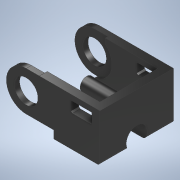
# Autodesk Inventor part: X-linear bearing shroud left half
Saved by Autodesk Inventor 2020.4 (Build 244396000, 396)
## iProperties
Created: 2021-02-25
Part Number: X-linear bearing shroud left half
Material: ABS Plastic
Document SubType Name: Modeling
Designer: AOB
Surface Area: 41.2852 cm^2
Density: 1.06 g/cm^3
Appearance: Glossy - Black
Mass: 4.81018 g
Volume: 4.53791 cm^3
Author: AOB
Autodesk Inventor part; units mm, degrees
ref_plane "YZ Plane" through (0, 0, 0) normal (1, 0, 0) x (0, 1, 0)
ref_plane "XZ Plane" through (0, 0, 0) normal (0, 1, 0) x (-1, 0, 0)
sketch "Sketch1" plane through (0, 0, 0) normal (0, 0, 1) x (1, 0, 0)
  line L0 (5.0224, 7.5) -> (28, 7.5)
  line L1 (5.0224, 7.5) -> (5.7962, 7.5)
  arc A0 (0, 7.5) -> (-0.0125, -7.5) centre (0, 0) ccw
  line L2 (5.0224, 7.5) -> (0, 7.5)
  line L3 (23.4991, -10.4606) -> (10.5, -10.4606)
  line L4 (10.5, -10.4606) -> (10.5, -7.5)
  line L5 (17.5, 1.4713) -> (24.5, 1.4713)
  line L6 (25, 1.9713) -> (25, 5.5001)
  line L7 (28, 7.5001) -> (28, -9.4606)
  line L8 (27, -10.4606) -> (23.4991, -10.4606)
  arc A1 (27, -10.4606) -> (28, -9.4606) centre (27, -9.4606) ccw
  line L9 (24.5, 1.4713) -> (25, 1.9713)
  line L10 (17.5, 1.4713) -> (17, 1.9713)
  line L11 (10.5, -7.5) -> (-0.0125, -7.5)
  line L12 (25, 5.5001) -> (17, 5.5001)
  line L13 (17, 7.5001) -> (17, 7.5)
  line L14 (17, 5.5001) -> (17, 1.9713)
  point P0 (25, 1.4713)
  point P1 (17, 1.4713)
  dimension "d58" = 1
  dimension "d70" = 28
  dimension "d71" = 17.5
  constraints: 30 end point, 6 perpendicular, 6 point on line, 4 horizontal, 4 point on circle, 3 tangent, 2 centre point, 1 coincident, 1 vertical
  measures "d58" radius of A1
  measures "d70" distance from line of L7 point (0, 0)
  measures "d71" distance between parallel lines of L7 L4
extrude "Extrusion1" add sketch "Sketch1" along normal blind 3
sketch "Sketch3" plane through (0, 0, 0) normal (0, 0, -1) x (-1, 0, 0)
  line L0 (-10.5, -10.4606) -> (-27, -10.4606)
  line L1 (-10.5, -7.5) -> (-10.5, -10.4606)
  arc A0 (-28, -9.4606) -> (-27, -10.4606) centre (-27, -9.4606) ccw
  line L2 (-28, -9.4606) -> (-28, 7.5)
  line L3 (-25, 5.5001) -> (-25, 1.9713)
  line L4 (-28, 7.5) -> (-25, 7.5)
  line L5 (-25, 5.5001) -> (-25, 7.5)
  line L6 (-25, 1.9713) -> (-24.5, 1.4713) projected
  line L7 (-25, 1.9713) -> (-25, -7.5)
  line L8 (-25, -7.5) -> (-10.5, -7.5)
  constraints: 16 end point, 2 perpendicular, 2 point on circle, 1 centre point, 1 point on line
extrude "Extrusion2" add sketch "Sketch3" along normal blind 11
ref_plane "Work Plane1" through (0, 0, -11) normal (0, 0, -1) x (-1, 0, 0)
sketch "Sketch4" plane through (25, 6.9501, 0) normal (-1, 0, 0) x (0, 0, 1)
  circle A0 centre (-11, -7.0106) radius 2.5
  line L0 (-11, -17.4106) -> (3, -17.4106) projected
  point P0 (0, -6.9501)
  point P1 (0, -17.4106)
  dimension "d22" = 5
  dimension "d73" = 10.4
  constraints: 1 centre point
  measures "d22" diameter of A0
  measures "d73" distance from line of L0 A0.centre
extrude "Extrusion3" add sketch "Sketch4" along normal blind 16
sketch "Sketch6" plane through (0, 0, 0) normal (0, 0, -1) x (-1, 0, 0)
  arc A0 (5.0124, 5.594) -> (0, 7.5) centre (0, -0.0439) ccw
  line L0 (-5.0224, 7.5) -> (-5.0224, 5.5851)
  circle A1 centre (0, -0.0439) radius 4.5
  circle A2 centre (0, -0.0439) radius 7.5439
  line L1 (-28, 7.5) -> (-5.0224, 7.5) projected
  line L2 (-5.0224, 7.5) -> (0, 7.5)
  point P0 (0, 0)
  point P1 (5.0224, 5.5902)
  point P2 (-17, 7.5)
  point P3 (0, 7.5)
  point P4 (5.0124, 5.594)
  dimension "d37" = 9
  constraints: 4 end point, 2 centre point, 2 coincident, 2 point on circle, 1 tangent, 4 other
  measures "d37" diameter of A1
extrude "Extrusion4" cut sketch "Sketch6" against normal mid plane 2 contours A2 A0 | A2 L0 L2 | A1
extrude "Extrusion5" cut sketch "Sketch6" against normal through all contours A1
mirror "Mirror4" about plane through (0, 0, -11) normal (0, 0, -1) of "Extrusion1", "Extrusion2", "Extrusion4", "Extrusion5"
sketch "Sketch7" plane through (25, -9.4606, 0) normal (1, 0, 0) x (0, 0, -1)
  line L0 (0, -1.0053) -> (22, -1.0053)
  circle A0 centre (11, 1.2078) radius 4
  point P0 (0, 9.4606)
  dimension "d49" = 8
  dimension "d72" = 2.2131
  constraints: 2 end point, 1 centre point
  measures "d49" diameter of A0
  measures "d72" distance from line of L0 A0.centre
extrude "Extrusion6" cut sketch "Sketch7" along normal through all both and the other way through all
body "Solid1"
